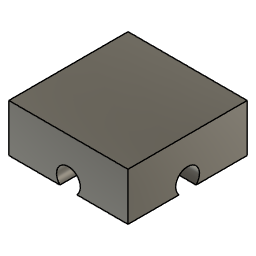
pääprojekti v11 (Autodesk Fusion 360 archive; units mm, degrees)
design "demopala narupidike"
Autodesk Fusion 360 part; units mm, degrees
sketch "Sketch1" plane through (0, 0, 0) normal (0, 0, 1) x (1, 0, 0)
  line L0 (12.5, 12.5) -> (-12.5, 12.5)
  line L1 (-12.5, 12.5) -> (-12.5, -12.5)
  line L2 (-12.5, -12.5) -> (12.5, -12.5)
  line L3 (12.5, -12.5) -> (12.5, 12.5)
  line L4 (12.5, 12.5) -> (-12.5, -12.5) construction
  line L5 (-12.5, 12.5) -> (12.5, -12.5) construction
  dimension "d1" = 25
  dimension "d2" = 25
  constraint horizontal L0
  constraint perpendicular L0 L1
  constraint parallel L0 L2
  constraint parallel L1 L3
  constraint coincident L4 origin
  constraint coincident L5 origin
  measures "d1" distance of L1.end L2.end
  measures "d2" distance of L0.end L1.end
extrude "Extrude1" add sketch "Sketch1" along normal blind 10
sketch "Sketch2" plane through (12.5, 0, 0) normal (1, 0, 0) x (0, 1, 0)
  line L0 (-12.5, 0) -> (12.5, 0)
  line L1 (12.5, 0) -> (12.5, 10)
  line L2 (12.5, 10) -> (-12.5, 10)
  line L3 (-12.5, 10) -> (-12.5, 0)
  circle A0 centre (0, 1.75) radius 2.5
  dimension "d5" = 5
  dimension "d6" = 1.75
  measures "d5" diameter of A0
  measures "d6" distance of origin A0.centre
sketch "Sketch3" plane through (0, -12.5, 0) normal (0, -1, 0) x (1, 0, 0)
  line L0 (-12.5, 0) -> (12.5, 0)
  line L1 (12.5, 0) -> (12.5, 10)
  line L2 (12.5, 10) -> (-12.5, 10)
  line L3 (-12.5, 10) -> (-12.5, 0)
  circle A0 centre (0, 1.75) radius 2.5
  dimension "d7" = 5
  dimension "d8" = 1.75
  measures "d7" diameter of A0
  measures "d8" distance of origin A0.centre
extrude "Extrude2" cut sketch "Sketch3" against normal blind 25 contours L0 A0 picked at (0.8618, 1.7195)
extrude "Extrude3" cut sketch "Sketch2" against normal blind 25 contours L0 A0 picked at (0.8341, 1.5065)
